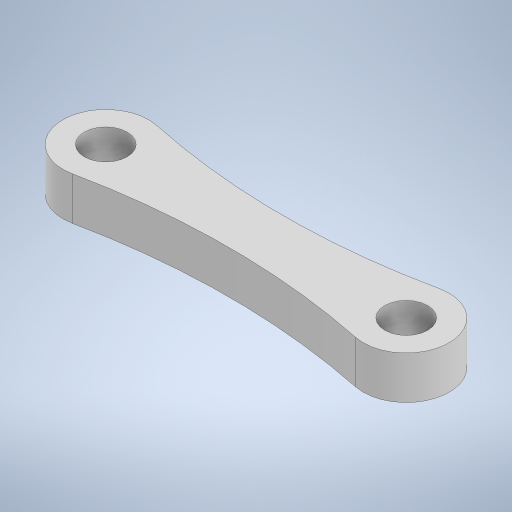
# Autodesk Inventor part: body-tail
Saved by Autodesk Inventor 2024 (Build 280153000, 153)
## iProperties
Created: 2023-10-17
Part Number: body-tail
Material: Generic
Document SubType Name: Modeling
Designer: Piter
Density: 1 g/cm^3
Appearance: Default
Author: Piter
Autodesk Inventor part; units mm, degrees
ref_plane "YZ Plane" through (0, 0, 0) normal (1, 0, 0) x (0, 1, 0)
ref_plane "XZ Plane" through (0, 0, 0) normal (0, 1, 0) x (-1, 0, 0)
ref_plane "XY Plane" through (0, 0, 0) normal (0, 0, 1) x (1, 0, 0)
sketch "Sketch1" plane through (0, 0, 0) normal (0, 1, 0) x (-1, 0, 0)
  line L0 (-15.1311, 4.4797) -> (19.8689, 4.4797)
  circle A0 centre (19.8689, 4.4797) radius 2.5
  circle A1 centre (-15.1311, 4.4797) radius 2.5
  circle A2 centre (-15.1311, 4.4797) radius 5
  circle A3 centre (19.8689, 4.4797) radius 5
  line L1 (2.3689, 4.4797) -> (2.3689, 1.3284)
  line L2 (2.3689, 1.3284) -> (2.3689, 4.4797)
  line L3 (2.3689, 4.4797) -> (2.3689, 7.6857)
  arc A4 (-14.1166, 9.3757) -> (18.8544, 9.3757) centre (2.3689, 88.9357) ccw
  arc A5 (18.8242, -0.4099) -> (-14.0864, -0.4099) centre (2.3689, -77.427) ccw
  point P0 (0, 0)
  point P1 (7.7903, 4.509)
  dimension "d0" = 35
  dimension "d1" = 5
  dimension "d2" = 5
  dimension "d3" = 10
  dimension "d4" = 10
  constraints: 10 point on circle, 8 end point, 6 centre point, 4 coincident, 4 tangent, 2 vertical, 1 collinear, 1 horizontal, 1 midpoint
  measures "d0" distance of L0.start L0.end
  measures "d1" diameter of A0
  measures "d2" diameter of A1
  measures "d3" diameter of A2
  measures "d4" diameter of A3
extrude "Extrusion1" add sketch "Sketch1" along normal blind 5
body "Solid1"
